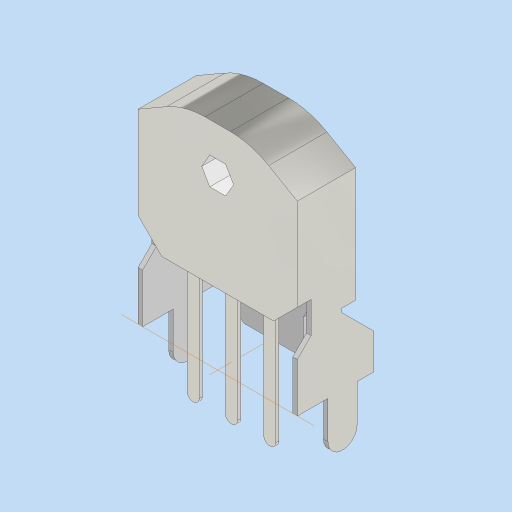
# Autodesk Inventor part: TTC_silver_rotary_encoder
Saved by Autodesk Inventor 2024 (Build 280153000, 153)
## iProperties
Created: 2025-05-06
Part Number: TTC_silver_rotary_encoder
Material: Generic
Document SubType Name: Modeling
Designer: XxPan
Density: 1 g/cm^3
Appearance: Default
Author: XxPan
Autodesk Inventor part; units mm, degrees
ref_plane "YZ Plane" through (0, 0, 0) normal (1, 0, 0) x (0, 1, 0)
ref_plane "XZ Plane" through (0, 0, 0) normal (0, 1, 0) x (-1, 0, 0)
sketch "Sketch1" plane through (0, 0, 0) normal (0, 0, 1) x (1, 0, 0)
  line L0 (-3.65, 4.6) -> (3.65, 4.6)
  line L1 (3.65, 4.6) -> (5.2, 6.15)
  line L2 (5.2, 6.15) -> (5.2, 12.15)
  line L3 (5.2, 12.15) -> (2.1689, 13.9)
  line L4 (2.1689, 13.9) -> (-2.1689, 13.9)
  line L5 (-2.1689, 13.9) -> (-5.2, 12.15)
  line L6 (-5.2, 12.15) -> (-5.2, 6.15)
  line L7 (-5.2, 6.15) -> (-3.65, 4.6)
  line L8 (0, -2.78) -> (0, 16.68) construction
  circle A0 centre (0, 11) radius 1.1
  line L9 (-7.28, 0) -> (7.28, 0) projected
  dimension "d42" = 2.2
  dimension "d43" = 10.4
  dimension "d44" = 9.3
  dimension "d45" = 45
  dimension "d46" = 45
  dimension "d47" = 6
  dimension "d48" = 7.3
  dimension "d49" = 2.9
  dimension "d50" = 11
  constraints: 16 end point, 2 horizontal alignment, 1 centre point, 1 horizontal, 1 parallel, 1 perpendicular, 1 point on line, 1 vertical, 2 other
  measures "d42" diameter of A0
  measures "d43" distance between parallel lines of L2 L6
  measures "d44" distance between parallel lines of L0 L4
  measures "d45" angle of L0 L7
  measures "d46" angle of L0 L1
  measures "d47" distance of L1.end L2.end
  measures "d48" distance of L0.start L0.end
  measures "d49" distance from line of L4 A0.centre
  measures "d50" distance from line of L9 A0.centre
extrude "Extrusion1" add sketch "Sketch1" against normal blind 3.8
fillet "Fillet1" radius 5 2 edges at (2.1689, 13.9, -1.9) (-2.1689, 13.9, -1.9)
ref_plane "Work Plane1" through (0, 0, -1) normal (0, 0, 1) x (1, 0, 0)
sketch "Sketch2" plane through (0, 0, -1) normal (0, 0, 1) x (1, 0, 0)
  line L0 (-0.4, 4.6) -> (-0.4, -3.1)
  line L1 (0.4, 4.6) -> (0.4, -3.1)
  arc A0 (-0.4, -3.1) -> (0.4, -3.1) centre (0, -3.1) ccw
  line L2 (0, -6.98) -> (0, 17.38) construction
  line L3 (-3.65, 4.6) -> (3.65, 4.6) projected
  line L4 (-7.28, 0) -> (7.28, 0) construction
  point P0 (0, 0)
  point P1 (0, -3.5)
  dimension "d8" = 0.8
  dimension "d51" = 3.5
  constraints: 4 end point, 3 point on circle, 2 point on line, 2 tangent, 2 vertical, 1 centre point, 1 other
  measures "d8" distance between parallel lines of L1 L0
extrude "Extrusion2" add sketch "Sketch2" along normal mid plane 0.2 fills toward (0.35, 0.75) open curves L1 A0 L0
pattern_linear "Rectangular Pattern1" count 2 spacing 2.5 along (1, 0, 0) count 2 spacing 2.5 along (-1, 0, 0) of "Extrusion2"
sketch "Sketch10" plane through (5.2, 6.15, 0) normal (1, 0, 0) x (0, 0, -1)
  line L0 (0, 0) -> (3.8, 0) projected
  line L1 (0.9, 0) -> (0.9, -2.05)
  line L2 (0.9, -2.05) -> (0, -2.95)
  line L3 (0, -2.95) -> (0, -6.15)
  line L4 (0, -6.15) -> (5, -6.15)
  line L5 (5, -6.15) -> (5, -3.85)
  line L6 (5, -3.85) -> (2.9, -1.75)
  line L7 (2.9, -1.75) -> (2.9, -1.5)
  line L8 (2.9, -1.5) -> (3.8, -1.5)
  line L9 (3.8, -1.5) -> (3.8, 0)
  line L10 (0, 0) -> (0, 6) projected
  line L11 (3.8, 6) -> (3.8, 0) projected
  line L12 (2, -6.15) -> (2, -8.6)
  line L13 (3.9, -6.15) -> (3.9, -8.6)
  arc A0 (2, -8.6) -> (3.9, -8.6) centre (2.95, -8.6) ccw
  dimension "d53" = 2
  dimension "d55" = 3.8
  dimension "d56" = 0.9
  dimension "d57" = 1.5
  dimension "d58" = 5
  dimension "d59" = 45
  dimension "d61" = 45
  dimension "d62" = 2.3
  dimension "d63" = 3.2
  dimension "d66" = 3.4
  dimension "d67" = 1.9
  dimension "d68" = 2
  constraints: 22 end point, 5 perpendicular, 3 point on line, 2 parallel, 2 point on circle, 2 tangent, 2 vertical, 1 centre point
  measures "d53" distance between parallel lines of L7 L1
  measures "d55" distance between parallel lines of L11 L10
  measures "d56" distance between parallel lines of L10 L1
  measures "d57" distance between parallel lines of L0 L8
  measures "d58" distance of L3.end L4.end
  measures "d59" angle of L5 L6
  measures "d61" angle of L3 L2
  measures "d62" distance of L4.end L5.end
  measures "d63" distance of L2.end L3.end
  measures "d67" distance between parallel lines of L12 L13
  measures "d68" distance between parallel lines of L3 L12
extrude "Extrusion8" add sketch "Sketch10" against normal blind 0.3
mirror "Mirror3" about plane through (0, 0, 0) normal (1, 0, 0) of "Extrusion8"
sketch "Sketch11" plane through (0, 0, -3.8) normal (0, 0, -1) x (-1, 0, 0)
  line L0 (-3.65, 4.6) -> (3.65, 4.6) projected
  line L1 (-3.25, 4.6) -> (-2.1, 2.3)
  line L2 (-2.1, 2.3) -> (-2.1, 0)
  line L3 (-2.1, 0) -> (2.1, 0)
  line L4 (2.1, 0) -> (2.1, 2.3)
  line L5 (2.1, 2.3) -> (3.25, 4.6)
  line L6 (0, -6.98) -> (0, 17.38) construction
  line L7 (7.28, 0) -> (-7.28, 0) construction
  point P0 (0, 0)
  dimension "d69" = 2.3
  dimension "d70" = 4.2
  dimension "d71" = 6.5
  constraints: 10 end point, 2 perpendicular, 2 point on line, 1 collinear, 1 horizontal alignment, 2 other
  measures "d69" distance of L3.end L4.end
  measures "d70" distance of L2.end L3.end
  measures "d71" distance of L5.end L1.start
extrude "Extrusion9" add sketch "Sketch11" against normal blind 0.3
chamfer "Chamfer1" distance 0.3 angle 45 2 edges at (-2.1, 0, -3.65) (2.1, 0, -3.65)
sketch "Sketch7" plane through (0, 0, -3.8) normal (0, 0, 1) x (1, 0, 0)
  circle A0 centre (0, 11) radius 1.75
  line L0 (0, -6.98) -> (0, 17.38) construction
  circle A1 centre (0, 11) radius 1.1 projected
  point P0 (0, 0)
  dimension "d32" = 3.5
  constraints: 1 centre point, 1 coincident, 1 point on line
  measures "d32" diameter of A0
extrude "Extrusion5" add sketch "Sketch7" against normal blind 0.6
sketch "Sketch9" plane through (0, 11, 0) normal (0, 0, -1) x (-1, 0, 0)
  line L0 (1.0392, 0) -> (0.5196, -0.9)
  line L1 (0.5196, -0.9) -> (-0.5196, -0.9)
  line L2 (-0.5196, -0.9) -> (-1.0392, 0)
  line L3 (-1.0392, 0) -> (-0.5196, 0.9)
  line L4 (-0.5196, 0.9) -> (0.5196, 0.9)
  line L5 (0.5196, 0.9) -> (1.0392, 0)
  circle A0 centre (0, 0) radius 1.1 projected
  point P0 (0, -11)
  dimension "d39" = 1.8
  constraints: 12 end point, 1 coincident, 13 other
  measures "d39" distance between parallel lines of L1 L4
extrude "Extrusion7" add sketch "Sketch9" along normal blind 2.4
equation "\"d56\" = -0.5 * d53 + 0.5 * d55"
body "Solid1"
